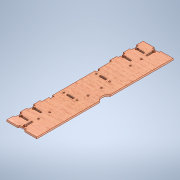
# Autodesk Inventor part: перед
Saved by Autodesk Inventor 2020 (Build 240168000, 168)
## iProperties
Created: 2025-01-17
Part Number: перед
Material: Древесина (дуб)
Document SubType Name: Modeling
Designer: frozj
Density: 0.76 g/cm^3
Appearance: Белый дуб — натуральный — с умеренным глянцем
Author: frozj
Autodesk Inventor part; units mm, degrees
ref_plane "YZ Plane" through (0, 0, 0) normal (1, 0, 0) x (0, 1, 0)
ref_plane "XZ Plane" through (0, 0, 0) normal (0, 1, 0) x (-1, 0, 0)
ref_plane "XY Plane" through (0, 0, 0) normal (0, 0, 1) x (1, 0, 0)
sketch "Эскиз1" plane through (0, 0, 0) normal (0, 1, 0) x (-1, 0, 0)
  line L0 (-28.5, -125) -> (28.5, -125)
  line L1 (28.5, -125) -> (28.5, 125)
  line L2 (28.5, 125) -> (-28.5, 125)
  line L3 (-28.5, 125) -> (-28.5, -125)
  line L4 (28.5, 125) -> (11.5, 125)
  line L5 (11.5, 125) -> (11.5, -125)
  line L6 (11.5, -125) -> (28.5, -125)
  line L7 (28.5, -125) -> (28.5, 125)
  line L8 (11.5, -125) -> (-8.5, -125)
  line L9 (-8.5, -125) -> (-8.5, 125)
  line L10 (-8.5, 125) -> (11.5, 125)
  line L11 (11.5, 125) -> (11.5, -125)
  line L12 (-8.5, 125) -> (-25.5, 125)
  line L13 (-25.5, 125) -> (-25.5, -125)
  line L14 (-25.5, -125) -> (-8.5, -125)
  line L15 (-8.5, -125) -> (-8.5, 125)
  line L16 (11.5, 14.5) -> (-8.5, 14.5)
  line L17 (-8.5, 14.5) -> (-8.5, -14.5)
  line L18 (-8.5, -14.5) -> (11.5, -14.5)
  line L19 (11.5, -14.5) -> (11.5, 14.5)
  line L20 (1.5, 0) -> (1.5, -14.5)
  line L21 (1.5, 0) -> (1.5, 14.5)
  line L22 (1.5, 0) -> (5.0733, 0)
  line L23 (1.5, 14.5) -> (1.5, 11.5)
  line L24 (28.5, 125) -> (25.5, 125)
  line L25 (25.5, 125) -> (25.5, -125)
  line L26 (25.5, -125) -> (28.5, -125)
  line L27 (28.5, -125) -> (28.5, 125)
  line L28 (28.5, 125) -> (25.5, 125)
  line L29 (25.5, 125) -> (25.5, 111)
  line L30 (25.5, 111) -> (28.5, 111)
  line L31 (28.5, 111) -> (28.5, 125)
  line L32 (25.5, 111) -> (28.5, 111)
  line L33 (28.5, 111) -> (28.5, 99)
  line L34 (28.5, 99) -> (25.5, 99)
  line L35 (25.5, 99) -> (25.5, 111)
  line L36 (25.5, 99) -> (28.5, 99)
  line L37 (28.5, 99) -> (28.5, 87)
  line L38 (28.5, 87) -> (25.5, 87)
  line L39 (25.5, 87) -> (25.5, 99)
  line L40 (25.5, 87) -> (28.5, 87)
  line L41 (28.5, 87) -> (28.5, 75)
  line L42 (28.5, 75) -> (25.5, 75)
  line L43 (25.5, 75) -> (25.5, 87)
  line L44 (25.5, 75) -> (28.5, 75)
  line L45 (28.5, 75) -> (28.5, 63)
  line L46 (28.5, 63) -> (25.5, 63)
  line L47 (25.5, 63) -> (25.5, 75)
  line L48 (28.5, 111) -> (28.5, 106.35)
  line L49 (28.5, 106.35) -> (8.5, 106.35)
  line L50 (8.5, 106.35) -> (8.5, 103.65)
  line L51 (8.5, 103.65) -> (28.5, 103.65)
  line L52 (28.5, 103.65) -> (28.5, 106.35)
  line L53 (25.5, 106.35) -> (22.5, 106.35)
  line L54 (22.5, 106.35) -> (22.5, 107.45)
  line L55 (22.5, 107.45) -> (25.5, 107.45)
  line L56 (25.5, 107.45) -> (25.5, 106.35)
  line L57 (22.5, 107.45) -> (20.6, 107.45)
  line L58 (20.6, 107.45) -> (20.6, 102.55)
  line L59 (20.6, 102.55) -> (22.5, 102.55)
  line L60 (22.5, 102.55) -> (22.5, 107.45)
  line L61 (28.5, 93) -> (26.2601, 93)
  line L62 (28.5, 79.65) -> (8.5, 79.65)
  line L63 (8.5, 82.35) -> (28.5, 82.35)
  line L64 (22.5, 78.55) -> (20.6, 78.55)
  line L65 (20.6, 78.55) -> (20.6, 83.45)
  line L66 (20.6, 83.45) -> (22.5, 83.45)
  line L67 (22.5, 83.45) -> (22.5, 78.55)
  line L68 (8.5, 79.65) -> (8.5, 82.35)
  line L69 (25.5, -111) -> (28.5, -111)
  line L70 (25.5, -87) -> (28.5, -87)
  line L71 (28.5, -75) -> (25.5, -75)
  line L72 (28.5, -63) -> (25.5, -63)
  line L73 (28.5, -106.35) -> (8.5, -106.35)
  line L74 (8.5, -106.35) -> (8.5, -103.65)
  line L75 (8.5, -103.65) -> (28.5, -103.65)
  line L76 (22.5, -107.45) -> (20.6, -107.45)
  line L77 (20.6, -107.45) -> (20.6, -102.55)
  line L78 (20.6, -102.55) -> (22.5, -102.55)
  line L79 (22.5, -102.55) -> (22.5, -107.45)
  line L80 (8.5, -82.35) -> (28.5, -82.35)
  line L81 (28.5, -79.65) -> (8.5, -79.65)
  line L82 (22.5, -83.45) -> (22.5, -78.55)
  line L83 (20.6, -78.55) -> (20.6, -83.45)
  line L84 (20.6, -83.45) -> (22.5, -83.45)
  line L85 (22.5, -78.55) -> (20.6, -78.55)
  line L86 (8.5, -79.65) -> (8.5, -82.35)
  line L87 (28.5, -87) -> (25.5, -87)
  line L88 (25.5, -99) -> (28.5, -99)
  line L89 (28.5, 125) -> (-28.5, 125)
  line L90 (-28.5, 125) -> (-28.5, 123)
  line L91 (-28.5, 123) -> (28.5, 123)
  line L92 (28.5, 123) -> (28.5, 125)
  line L93 (28.5, 123) -> (8.5, 123)
  line L94 (8.5, 123) -> (8.5, 120)
  line L95 (8.5, 120) -> (28.5, 120)
  line L96 (28.5, 120) -> (28.5, 123)
  line L97 (8.5, 120) -> (-3.5, 120)
  line L98 (-3.5, 120) -> (-3.5, 123)
  line L99 (-3.5, 123) -> (8.5, 123)
  line L100 (8.5, 123) -> (8.5, 120)
  line L101 (8.5, 123) -> (3.85, 123)
  line L102 (3.85, 123) -> (1.15, 123)
  line L103 (1.15, 123) -> (1.15, 103)
  line L104 (1.15, 103) -> (3.85, 103)
  line L105 (3.85, 103) -> (3.85, 123)
  line L106 (1.15, 120) -> (0.05, 120)
  line L107 (0.05, 120) -> (0.05, 117)
  line L108 (0.05, 117) -> (1.15, 117)
  line L109 (1.15, 117) -> (1.15, 120)
  line L110 (0.05, 117) -> (4.95, 117)
  line L111 (4.95, 117) -> (4.95, 115.1)
  line L112 (4.95, 115.1) -> (0.05, 115.1)
  line L113 (0.05, 115.1) -> (0.05, 117)
  line L114 (-28.5, -123) -> (28.5, -123)
  line L115 (8.5, -123) -> (8.5, -120)
  line L116 (8.5, -120) -> (28.5, -120)
  line L117 (8.5, -120) -> (-3.5, -120)
  line L118 (-3.5, -120) -> (-3.5, -123)
  line L119 (1.15, -123) -> (1.15, -103)
  line L120 (1.15, -103) -> (3.85, -103)
  line L121 (3.85, -103) -> (3.85, -123)
  line L122 (0.05, -117) -> (1.15, -117)
  line L123 (0.05, -117) -> (4.95, -117)
  line L124 (4.95, -117) -> (4.95, -115.1)
  line L125 (4.95, -115.1) -> (0.05, -115.1)
  line L126 (0.05, -115.1) -> (0.05, -117)
  line L127 (0, 0) -> (0, -36)
  line L128 (0, 0) -> (0, 47)
  line L129 (0, 47) -> (28.5, 47)
  line L130 (0, -36) -> (28.5, -36)
  line L131 (28.5, 47) -> (25.5, 47)
  line L132 (25.5, 47) -> (25.5, 45.5)
  line L133 (25.5, 45.5) -> (28.5, 45.5)
  line L134 (28.5, 45.5) -> (28.5, 47)
  line L135 (25.5, 45.5) -> (22.5, 45.5)
  line L136 (22.5, 45.5) -> (22.5, 48.5)
  line L137 (22.5, 48.5) -> (25.5, 48.5)
  line L138 (25.5, 48.5) -> (25.5, 45.5)
  line L139 (28.5, -36) -> (25.5, -36)
  line L140 (25.5, -36) -> (25.5, -34.5)
  line L141 (25.5, -34.5) -> (28.5, -34.5)
  line L142 (28.5, -34.5) -> (28.5, -36)
  line L143 (25.5, -34.5) -> (22.5, -34.5)
  line L144 (22.5, -34.5) -> (22.5, -37.5)
  line L145 (22.5, -37.5) -> (25.5, -37.5)
  line L146 (25.5, -37.5) -> (25.5, -34.5)
  line L147 (25.5, 0) -> (13.5, 0)
  line L148 (25.5, 20) -> (25.5, 0)
  line L149 (25.5, 0) -> (13.5, 0)
  line L150 (25.5, -20) -> (25.5, 0)
  line L151 (0, 0) -> (0, -47)
  line L152 (25.5, 0) -> (13.5, 0)
  line L153 (13.5, 0) -> (13.5, 29.5)
  line L154 (25.5, 29.5) -> (25.5, 0)
  line L155 (13.5, 29.5) -> (13.5, 28)
  line L156 (13.5, 28) -> (25.5, 28)
  line L157 (25.5, 28) -> (25.5, 29.5)
  line L158 (25.5, 28) -> (13.5, 28)
  line L159 (13.5, 28) -> (13.5, 31)
  line L160 (13.5, 31) -> (25.5, 31)
  line L161 (25.5, 31) -> (25.5, 28)
  line L162 (13.5, 31) -> (1.5, 31)
  line L163 (1.5, 31) -> (1.5, 28)
  line L164 (1.5, 28) -> (13.5, 28)
  line L165 (13.5, 28) -> (13.5, 31)
  line L166 (1.5, 31) -> (-10.5, 31)
  line L167 (-10.5, 31) -> (-10.5, 28)
  line L168 (-10.5, 28) -> (1.5, 28)
  line L169 (1.5, 28) -> (1.5, 31)
  circle A0 centre (19.5, 29.5) radius 1.5
  circle A1 centre (-4.5, 29.5) radius 1.5
  line L170 (11.5, -125) -> (11.5, 125)
  line L171 (13.5, -28) -> (25.5, -28)
  line L172 (13.5, -28) -> (13.5, -31)
  line L173 (13.5, -31) -> (25.5, -31)
  line L174 (13.5, -31) -> (1.5, -31)
  line L175 (1.5, -31) -> (1.5, -28)
  line L176 (1.5, -28) -> (13.5, -28)
  line L177 (1.5, -31) -> (-10.5, -31)
  line L178 (-10.5, -31) -> (-10.5, -28)
  line L179 (-10.5, -28) -> (1.5, -28)
  circle A2 centre (19.5, -29.5) radius 1.5
  circle A3 centre (-4.5, -29.5) radius 1.5
  line L180 (-25.5, 0) -> (-7, 0)
  line L181 (-7, 0) -> (-7, 12)
  line L182 (-7, 12) -> (-25.5, 12)
  line L183 (-25.5, 12) -> (-25.5, 0)
  circle A4 centre (-7, 12) radius 1.5
  circle A5 centre (-7, -12) radius 1.5
  line L184 (22.5, -36) -> (25.5, -36)
  line L185 (25.5, -36) -> (25.5, -39)
  line L186 (25.5, -39) -> (22.5, -39)
  line L187 (22.5, -39) -> (22.5, -36)
  line L188 (22.5, -36) -> (25.5, -36)
  line L189 (25.5, -36) -> (25.5, -33)
  line L190 (25.5, -33) -> (22.5, -33)
  line L191 (22.5, -33) -> (22.5, -36)
  line L192 (22.5, 47) -> (25.5, 47)
  line L193 (25.5, 47) -> (25.5, 50)
  line L194 (25.5, 50) -> (22.5, 50)
  line L195 (22.5, 50) -> (22.5, 47)
  line L196 (22.5, 47) -> (25.5, 47)
  line L197 (25.5, 47) -> (25.5, 44)
  line L198 (25.5, 44) -> (22.5, 44)
  line L199 (22.5, 44) -> (22.5, 47)
  line L200 (1.5, 0) -> (97.5, 0) construction
  line L201 (1.5, 0) -> (1.5, 93)
  line L202 (1.5, 0) -> (94.5, 0) construction
  circle A6 centre (1.5, 93) radius 1.5
  line L203 (1.5, 93) -> (1.5, 73)
  circle A7 centre (1.5, 73) radius 1.5
  circle A8 centre (1.5, -93) radius 1.5
  circle A9 centre (1.5, -73) radius 1.5
  line L204 (-22.5, -10) -> (-28.5, -10)
  line L205 (-28.5, -10) -> (-28.5, 10)
  line L206 (-28.5, 10) -> (-22.5, 10)
  line L207 (-22.5, 10) -> (-22.5, -10)
  line L208 (-22.5, -10) -> (-28.5, 10) construction
  line L209 (-28.5, -10) -> (-22.5, 10) construction
  arc A10 (-25.5, -10) -> (-25.5, 10) centre (-32.1332, 0) ccw
  point P0 (28.5, -111)
  point P1 (25.5, -111)
  point P2 (25.5, -106.35)
  point P3 (22.5, -106.35)
  point P4 (20.6, -106.35)
  point P5 (20.6, -103.65)
  point P6 (22.5, -103.65)
  point P7 (25.5, -103.65)
  point P8 (28.5, -87)
  point P9 (25.5, -87)
  point P10 (25.5, -82.35)
  point P11 (22.5, -82.35)
  point P12 (20.6, -82.35)
  point P13 (20.6, -79.65)
  point P14 (22.5, -79.65)
  point P15 (25.5, -79.65)
  point P16 (25.5, -75)
  point P17 (28.5, -75)
  point P18 (28.5, -63)
  point P19 (25.5, -63)
  point P20 (25.5, 79.65)
  point P21 (22.5, 79.65)
  point P22 (20.6, 79.65)
  point P23 (20.6, 82.35)
  point P24 (22.5, 82.35)
  point P25 (25.5, 82.35)
  point P26 (25.5, 103.65)
  point P27 (22.5, 103.65)
  point P28 (20.6, 103.65)
  point P29 (20.6, 106.35)
  point P30 (1.15, -120)
  point P31 (1.15, -117)
  point P32 (1.15, -115.1)
  point P33 (3.85, -115.1)
  point P34 (3.85, -117)
  point P35 (3.85, -120)
  point P36 (28.5, 123)
  point P37 (3.85, 120)
  point P38 (3.85, 117)
  point P39 (3.85, 115.1)
  point P40 (1.15, 115.1)
  point P41 (1.15, 117)
  point P42 (-28.5, -123)
  point P43 (25.5, 48.5)
  point P44 (25.5, -37.5)
  point P45 (-25.5, 123)
  point P46 (-25.5, -123)
  dimension "d0" = 57
  dimension "d1" = 250
  dimension "d2" = 17
  dimension "d3" = 20
  dimension "d4" = 17
  dimension "d5" = 29
  dimension "d6" = 3
  dimension "d8" = 3
  dimension "d9" = 14
  dimension "d10" = 12
  dimension "d11" = 12
  dimension "d12" = 12
  dimension "d13" = 12
  dimension "d14" = 4.65
  dimension "d15" = 20
  dimension "d16" = 2.7
  dimension "d17" = 3
  dimension "d18" = 1.1
  dimension "d19" = 1.9
  dimension "d20" = 4.9
  dimension "d23" = 2
  dimension "d24" = 20
  dimension "d25" = 3
  dimension "d26" = 12
  dimension "d27" = 4.65
  dimension "d28" = 2.7
  dimension "d29" = 20
  dimension "d30" = 1.1
  dimension "d31" = 3
  dimension "d32" = 4.9
  dimension "d33" = 1.9
  dimension "d34" = 2
  dimension "d35" = 36
  dimension "d37" = 1.5
  dimension "d38" = 3
  dimension "d39" = 3
  dimension "d40" = 1.5
  dimension "d41" = 3
  dimension "d42" = 47
  dimension "d52" = 12
  dimension "d53" = 29.5
  dimension "d54" = 1.5
  dimension "d55" = 3
  dimension "d56" = 12
  dimension "d57" = 12
  dimension "d58" = 3
  dimension "d59" = 18.5
  dimension "d60" = 12
  dimension "d61" = 3
  dimension "d62" = 3
  dimension "d63" = 3
  dimension "d64" = 3
  dimension "d65" = 3
  dimension "d68" = 93
  dimension "d69" = 90
  dimension "d70" = 3
  dimension "d71" = 20
  dimension "d72" = 3
  dimension "d73" = 20
  dimension "d74" = 12
  constraints: 418 end point, 70 symmetric about line, 67 parallel, 40 horizontal, 37 perpendicular, 26 point on line, 11 centre point, 10 midpoint, 4 vertical, 3 coincident, 2 point on circle, 16 other
  measures "d0" distance of L2.end L1.end
  measures "d1" distance of L1.end L0.end
  measures "d2" distance of L6.end L5.end
  measures "d3" distance of L9.end L10.end
  measures "d4" distance of L14.end L13.end
  measures "d5" distance of L17.end L16.end
  measures "d6" distance of L21.end L23.end
  measures "d8" distance of L26.end L26.start
  measures "d9" distance of L29.end L28.end
  measures "d10" distance of L32.end L33.end
  measures "d11" distance of L36.end L37.end
  measures "d12" distance of L40.end L41.end
  measures "d13" distance of L44.end L45.end
  measures "d14" distance of L32.end L48.end
  measures "d15" distance of L51.end L50.end
  measures "d16" distance of L50.end L49.end
  measures "d17" distance of L54.end L55.end
  measures "d18" distance of L53.end L54.end
  measures "d19" distance of L59.end L58.end
  measures "d20" distance of L58.end L57.end
  measures "d23" distance of L90.end L89.end
  measures "d24" distance of L95.end L94.end
  measures "d25" distance of L94.end L93.end
  measures "d26" distance of L98.end L99.end
  measures "d27" distance of L99.end L101.end
  measures "d28" distance of L104.end L103.end
  measures "d29" distance of L103.end L102.end
  measures "d30" distance of L108.end L107.end
  measures "d31" distance of L107.end L106.end
  measures "d32" distance of L111.end L112.end
  measures "d33" distance of L110.end L111.end
  measures "d34" distance between parallel lines of L0 L114
  measures "d35" distance of L127.start L127.end
  measures "d37" distance of L132.end L131.end
  measures "d38" distance of L136.end L137.end
  measures "d39" distance of L135.end L136.end
  measures "d40" distance of L139.end L140.end
  measures "d41" distance of L144.end L143.end
  measures "d42" distance from line of L127.start L129
  measures "d52" distance of L153.end L154.start
  measures "d53" distance of L152.end L153.end
  measures "d54" distance of L155.end L155.start
  measures "d55" distance of L158.end L159.end
  measures "d56" distance of L164.end L163.end
  measures "d57" distance of L168.end L167.end
  measures "d58" diameter of A0
  measures "d59" distance of L182.end L181.end
  measures "d60" distance of L181.end L180.end
  measures "d61" diameter of A4
  measures "d62" distance of L184.end L185.end
  measures "d63" distance of L189.end L188.end
  measures "d64" distance of L193.end L192.end
  measures "d65" distance of L196.end L197.end
  measures "d68" distance of L20.start L201.end
  measures "d69" angle of L202 L201
  measures "d70" diameter of A6
  measures "d71" distance of L203.start L203.end
  measures "d72" diameter of A7
  measures "d73" distance of L204.end L205.end
  measures "d74" radius of A10
extrude "Выдавливание1" add sketch "Эскиз1" along normal blind 3 contours L13 L204 L207 A10 L180 L9 L179 L178 L177 L114 | L9 L177 L127 L130 L5 L81 L86 L80 L75 L74 L73 L116 L117 L121 L123 L124 L125 L120 L119 L126 L122 L118 L114 | A10 L207 L204 | L114 L115 L116 L5 | L5 L116 L25 L114 | L177 L178 L179 L9 | L9 L179 A3 L177 | L13 L182 L9 L180 A10 L207 L206 | L206 L207 A10 | L25 L116 L1 L114 | L5 L73 L77 L76 L79 L25 L116 | L9 L18 L127 L179 | A3 L179 L127 L177 | L91 L9 L166 L167 L168 L182 L13 | L25 L69 L1 L116 | L9 L180 L181 A4 L16 L128 L127 L18 | L177 L174 L5 L130 L127 | L127 L179 L175 L177 | L9 A4 L181 L180 | L91 L98 L97 L107 L113 L112 L103 L104 L105 L111 L110 L95 L5 L49 L50 L51 L63 L68 L62 L129 L128 L166 L9 | L5 L80 L83 L84 L82 L25 L75 L79 L78 L77 | L127 L128 L16 L21 L20 L18 | L18 L5 L176 L179 L127 | L166 A1 L168 L9 | L9 L168 L167 L166 | L9 L168 L128 L16 | L20 L21 L16 L5 L18 | L130 L144 L187 L186 L25 L81 L82 L85 L83 L5 | L5 L174 L173 L25 L190 L191 L144 L130 | L166 L128 L168 A1 | L128 L168 L201 L16 | L5 L164 L153 L147 L25 L171 L176 | L172 L171 A2 L173 | L91 L25 L95 L5 | L5 L95 L94 L91 | L166 L163 L168 L128 | L128 L129 L201 L166 | L103 L108 L107 L97 | L201 L164 L5 L16 | L25 L70 L1 L88 | A2 L171 L25 L173 | L91 L1 L95 L25 | L95 L25 L55 L57 L58 L49 L5 | L201 L129 L5 L162 | L95 L1 L30 L25 | L5 L129 L136 L199 L198 L25 L160 L162 | L156 L25 L147 L153 | L153 L159 L160 A0 L156 | L1 L71 L25 L72 | L51 L58 L59 L60 L25 L63 L67 L66 L65 L5 | L5 L62 L65 L64 L67 L25 L194 L195 L136 L129 | A0 L160 L25 L156 | L25 L49 L54 L55 | L46 L25 L42 L1 | L1 L38 L25 L34
